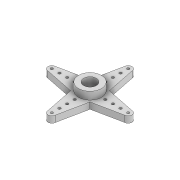
# Autodesk Inventor part: 90Horn
Saved by Autodesk Inventor 2022 (Build 260153000, 153)
## iProperties
Created: 2022-03-09
Part Number: 90Horn
Material: Generic
Document SubType Name: Modeling
Designer: piers
Density: 1 g/cm^3
Appearance: Default
Author: piers
Autodesk Inventor part; units mm, degrees
ref_plane "YZ Plane" through (0, 0, 0) normal (1, 0, 0) x (0, 1, 0)
ref_plane "XZ Plane" through (0, 0, 0) normal (0, 1, 0) x (-1, 0, 0)
ref_plane "XY Plane" through (0, 0, 0) normal (0, 0, 1) x (1, 0, 0)
sketch "Sketch1" plane through (0, 0, 0) normal (0, 1, 0) x (-1, 0, 0)
  circle A0 centre (0, 0) radius 4.5
  line L0 (0, 0) -> (0, -15)
  circle A1 centre (0, -15) radius 0.5
  circle A2 centre (0, -15) radius 1.5
  line L1 (4.3151, -1.2768) -> (1.4994, -15.0417)
  line L2 (-4.3151, -1.2768) -> (-1.4994, -15.0417)
  circle A3 centre (0, -6) radius 0.5
  circle A4 centre (0, -9) radius 0.5
  circle A5 centre (0, -12) radius 0.5
  line L3 (0, 0) -> (-1.4994, 0)
  circle A6 centre (0, 15) radius 0.5
  circle A7 centre (0, 15) radius 1.5
  line L4 (4.3151, 1.2768) -> (1.4994, 15.0417)
  line L5 (-4.3151, 1.2768) -> (-1.4994, 15.0417)
  circle A8 centre (0, 6) radius 0.5
  circle A9 centre (0, 9) radius 0.5
  circle A10 centre (0, 12) radius 0.5
  circle A11 centre (0, 0) radius 2.5
  circle A12 centre (-6, 0) radius 0.5
  circle A13 centre (-9, 0) radius 0.5
  circle A14 centre (-12, 0) radius 0.5
  circle A15 centre (-15, 0) radius 0.5
  circle A16 centre (-15, 0) radius 1.5
  line L6 (-1.2768, -4.3151) -> (-15.0417, -1.4994)
  line L7 (-1.2768, 4.3151) -> (-15.0417, 1.4994)
  circle A17 centre (0, 6) radius 0.5
  circle A18 centre (0, 9) radius 0.5
  circle A19 centre (0, 12) radius 0.5
  circle A20 centre (0, 15) radius 0.5
  circle A21 centre (0, 15) radius 1.5
  line L8 (-4.3151, 1.2768) -> (-1.4994, 15.0417)
  line L9 (4.3151, 1.2768) -> (1.4994, 15.0417)
  circle A22 centre (6, 0) radius 0.5
  circle A23 centre (9, 0) radius 0.5
  circle A24 centre (12, 0) radius 0.5
  circle A25 centre (15, 0) radius 0.5
  circle A26 centre (15, 0) radius 1.5
  line L10 (1.2768, 4.3151) -> (15.0417, 1.4994)
  line L11 (1.2768, -4.3151) -> (15.0417, -1.4994)
  point P0 (3.7991, -3.7991)
  point P1 (3.7991, 3.7991)
  point P2 (-3.7991, 3.7991)
  point P3 (-15.0417, 1.4994)
  point P4 (-3.7991, -3.7991)
  dimension "d0" = 9
  dimension "d3" = 3
  dimension "d1" = 15
  dimension "d2" = 1
  dimension "d4" = 1
  dimension "d5" = 1
  dimension "d6" = 1
  dimension "d8" = 3
  dimension "d9" = 3
  dimension "d10" = 3
  dimension "d13" = 5
  dimension "d18" = 360
  constraints: 24 end point, 21 centre point, 12 coincident, 12 symmetric about line, 3 point on line, 2 horizontal, 1 vertical, 91 other
  measures "d1" distance of L0.start L0.end
  measures "d2" diameter of A1
  measures "d4" diameter of A3
  measures "d5" diameter of A4
  measures "d6" diameter of A5
  measures "d8" distance of L0.end A5.centre
  measures "d9" distance of A4.centre A5.centre
  measures "d10" distance of A3.centre A4.centre
  measures "d13" diameter of A11
extrude "Extrusion1" add sketch "Sketch1" along normal blind 2.5 contours A0 L4 L10 A26 L11 L1 | A0 L10 L4 | L1 L11 A0 | A0 L7 L5 A7 L4 L10 | L11 L1 A2 L0 A5 A4 A3 A0 | A0 L5 L7 | A7 | A26 | L0 A3 A4 A5 A2 L2 L6 A0 | A2 | A0 L2 L6 A16 L7 L5 | L6 L2 A0 | A16
extrude "Extrusion2" add sketch "Sketch1" along normal blind 5.5 contours A0
body "Solid1"
